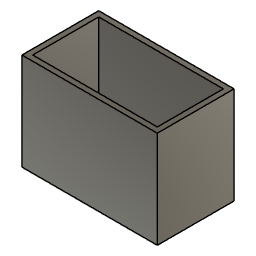
MotorHousingSkull v1 (Autodesk Fusion 360 design; units mm, degrees)
Autodesk Fusion 360 part; units mm, degrees
sketch "Sketch1" plane through (0, 0, 0) normal (0, 0, 1) x (1, 0, 0)
  line L0 (0, 0) -> (25.1, 0)
  line L1 (25.1, 0) -> (25.1, 14.23)
  line L2 (25.1, 14.23) -> (0, 14.23)
  line L3 (0, 14.23) -> (0, 0)
  dimension "d1" = 25.1
  dimension "d2" = 14.23
  constraint horizontal L0
  constraint vertical L1
  constraint horizontal L2
  constraint vertical L3
  constraint coincident L0.start L3.end
  measures "d1" distance of L0.start L0.end
  measures "d2" distance of L0.end L1.end
extrude "Extrude1" add sketch "Sketch1" along normal blind 18
shell "Shell1" thickness 1 removed faces 1 at (8.3667, 9.4867, 18)
sketch "Sketch2" plane through (0, 0, 1) normal (0, 0, 1) x (-1, 0, 0)
  line L0 (-1, -13.23) -> (-1, -1)
  line L1 (-1, -1) -> (-24.1, -1)
  line L2 (-24.1, -1) -> (-24.1, -13.23)
  line L3 (-24.1, -13.23) -> (-1, -13.23)
  line L4 (-1, -2.9885) -> (-3.56, -2.9885)
  line L5 (-3.56, -2.9885) -> (-3.56, -10.6185)
  line L6 (-3.56, -10.6185) -> (-1, -10.6185)
  line L7 (-1, -10.6185) -> (-1, -2.9885)
  line L8 (-24.1, -3.0078) -> (-21.54, -3.0078)
  line L9 (-21.54, -3.0078) -> (-21.54, -10.6378)
  line L10 (-21.54, -10.6378) -> (-24.1, -10.6378)
  line L11 (-24.1, -10.6378) -> (-24.1, -3.0078)
  dimension "d6" = 2.56
  dimension "d7" = 7.63
  dimension "d8" = 7.63
  dimension "d9" = 2.56
  constraint horizontal L4
  constraint vertical L5
  constraint horizontal L6
  constraint vertical L7
  constraint coincident L0 L4.start
  constraint horizontal L8
  constraint vertical L9
  constraint horizontal L10
  constraint vertical L11
  constraint coincident L2 L8.start
  measures "d6" distance of L5.end L6.end
  measures "d7" distance of L4.start L6.end
  measures "d8" distance of L8.end L9.end
  measures "d9" distance of L9.end L10.end
extrude "Extrude2" cut sketch "Sketch2" against normal blind 5 contours L0 L4 L5 L6 L7 | L2 L8 L9 L10 L11
